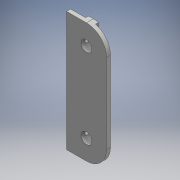
# Autodesk Inventor part: gap filler y axis
Saved by Autodesk Inventor 2016 (Build 200138000, 138)
## iProperties
Created: 2016-04-24
Part Number: gap filler y axis
Material: Generic
Document SubType Name: Modeling
Designer: Erwin
Density: 1 g/cm^3
Appearance: Default
Author: Erwin
Autodesk Inventor part; units mm, degrees
ref_plane "YZ Plane" through (0, 0, 0) normal (1, 0, 0) x (0, 1, 0)
ref_plane "XZ Plane" through (0, 0, 0) normal (0, 1, 0) x (-1, 0, 0)
ref_plane "XY Plane" through (0, 0, 0) normal (0, 0, 1) x (1, 0, 0)
sketch "Sketch1" plane through (0, 0, 0) normal (0, 1, 0) x (-1, 0, 0)
  line L0 (0, 0) -> (20, 0)
  line L1 (20, 0) -> (20, -60)
  line L2 (20, -60) -> (0, -60)
  line L3 (0, -60) -> (0, 0)
  dimension "d0" = 20
  dimension "d1" = 60
  constraints: 8 end point, 2 parallel, 1 horizontal, 1 perpendicular
  measures "d0" distance of L1.end L2.end
  measures "d1" distance of L0.end L1.end
extrude "Extrusion1" add sketch "Sketch1" along normal blind 2
sketch "Sketch2" plane through (0, 2, 0) normal (0, 1, 0) x (1, 0, 0)
  line L0 (0, 60) -> (-20, 60) projected
  line L1 (-7.5, 0) -> (-12.5, 0)
  line L2 (-12.5, 0) -> (-12.5, 60)
  line L3 (-12.5, 60) -> (-7.5, 60)
  line L4 (-7.5, 60) -> (-7.5, 0)
  line L5 (-7.5, 0) -> (-12.5, 60) construction
  line L6 (-12.5, 0) -> (-7.5, 60) construction
  point P0 (0, 0)
  point P1 (-10, 30)
  dimension "d4" = 5
  constraints: 12 end point, 2 midpoint, 2 parallel, 1 horizontal, 1 perpendicular, 1 point on line
  measures "d4" distance of L2.end L3.end
extrude "Extrusion2" add sketch "Sketch2" along normal blind 1.5
fillet "Fillet1" radius 10 2 edges at (0, 1, 0) (0, 1, -60)
sketch "Sketch3" plane through (0, 0, 0) normal (0, -1, 0) x (1, 0, 0)
  point P0 (0, 0)
  point P1 (-10, -50)
  point P2 (-10, -10)
hole "Hole1" at (-10, 0, -50) at (-10, 0, -10) direction (0, 1, 0) diameter 5.5 end through all
body "Solid1"
